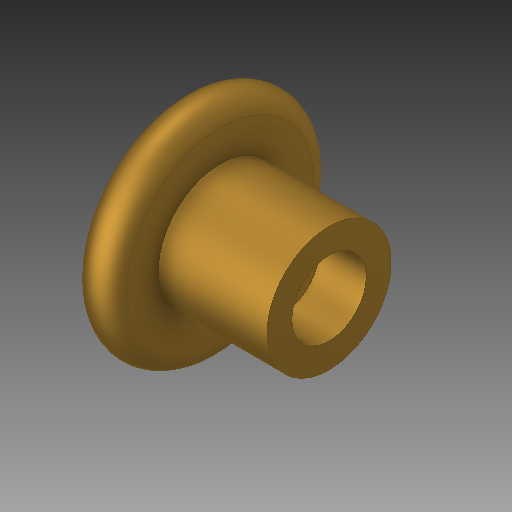
# Autodesk Inventor part: Rivet
Saved by Autodesk Inventor 2019 (Build 230136000, 136)
## iProperties
Company: Autodesk Inc.
Created: 2017-07-17
Part Number: Rivet
Material: Brass, Soft Yellow
Document SubType Name: Modeling
Designer: Autodesk Inc.
Density: 8.47 g/cm^3
Appearance: Brass - Satin
Mass: 0.0864071 g
Surface Area: 0.381623 cm^2
Volume: 0.0102015 cm^3
Author: Inventor
Autodesk Inventor part; units mm, degrees
ref_plane "YZ Plane" through (0, 0, 0) normal (1, 0, 0) x (0, 1, 0)
ref_plane "XZ Plane" through (0, 0, 0) normal (0, 1, 0) x (-1, 0, 0)
ref_plane "XY Plane" through (0, 0, 0) normal (0, 0, 1) x (1, 0, 0)
sketch "Sketch1" plane through (0, 0, 0) normal (0, 0, 1) x (1, 0, 0)
  arc A0 (0.6, 1.5) -> (0, 1.5) centre (0.3, 1.5) ccw
  line L0 (0, 0) -> (0, 1.5)
  line L1 (0.6, 1) -> (2.35, 1)
  line L2 (0.6, 1.5) -> (0.6, 1)
  line L3 (1.5964, 0.6) -> (2.35, 0.6)
  line L4 (2.35, 1) -> (2.35, 0.6)
  line L5 (1.25, 0) -> (1.5964, 0.6)
  line L6 (0, 0) -> (1.25, 0)
  point P0 (0, 1)
  dimension "d1" = 0.6
  dimension "d3" = 1.75
  dimension "d6" = 1.25
  dimension "d8" = 120
  dimension "d9" = 1.2
  dimension "d10" = 2
  dimension "d11" = 3
  constraints: 14 end point, 3 horizontal, 3 vertical, 2 point on circle, 1 centre point, 1 horizontal alignment, 1 point on line, 1 tangent, 1 vertical alignment
  measures "d1" diameter of A0
  measures "d3" distance from line of L1.end L2
  measures "d6" distance of L0.start L5.start
  measures "d8" angle of L6 L5
  measures "d9" diameter of L3 L6
  measures "d10" diameter of L1 L6
  measures "d11" diameter of A0.centre L6
revolve "Revolution1" add sketch "Sketch1" angle 360 about axis through (0, 0, 0) along (1, 0, 0)
body "Solid1"
